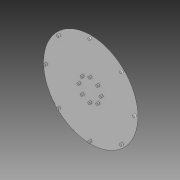
# Autodesk Inventor part: Deskcap
Saved by Autodesk Inventor 2020 (Build 240168000, 168)
## iProperties
Created: 2021-07-12
Part Number: Deskcap
Material: Generic
Document SubType Name: Modeling
Designer: DDeGo
Density: 1 g/cm^3
Appearance: Default
Author: DDeGo
Autodesk Inventor part; units mm, degrees
ref_plane "YZ Plane" through (0, 0, 0) normal (1, 0, 0) x (0, 1, 0)
ref_plane "XZ Plane" through (0, 0, 0) normal (0, 1, 0) x (-1, 0, 0)
ref_plane "XY Plane" through (0, 0, 0) normal (0, 0, 1) x (1, 0, 0)
sketch "Sketch1" plane through (0, 0, 0) normal (0, 0, 1) x (1, 0, 0)
  circle A0 centre (20, 0) radius 2.25
  circle A1 centre (80, 0) radius 2.25
  circle A2 centre (0, 0) radius 85
  line L0 (0, 0) -> (20, 0) construction
  line L1 (20, 0) -> (80, 0) construction
  circle A3 centre (14.1421, 14.1421) radius 2.25
  circle A4 centre (56.5685, 56.5685) radius 2.25
  line L2 (0, 0) -> (14.1421, 14.1421) construction
  line L3 (14.1421, 14.1421) -> (56.5685, 56.5685) construction
  circle A5 centre (0, 20) radius 2.25
  circle A6 centre (0, 80) radius 2.25
  line L4 (0, 0) -> (0, 20) construction
  line L5 (0, 20) -> (0, 80) construction
  circle A7 centre (-14.1421, 14.1421) radius 2.25
  circle A8 centre (-56.5685, 56.5685) radius 2.25
  line L6 (0, 0) -> (-14.1421, 14.1421) construction
  line L7 (-14.1421, 14.1421) -> (-56.5685, 56.5685) construction
  circle A9 centre (-20, 0) radius 2.25
  circle A10 centre (-80, 0) radius 2.25
  line L8 (0, 0) -> (-20, 0) construction
  line L9 (-20, 0) -> (-80, 0) construction
  circle A11 centre (-14.1421, -14.1421) radius 2.25
  circle A12 centre (-56.5685, -56.5685) radius 2.25
  line L10 (0, 0) -> (-14.1421, -14.1421) construction
  line L11 (-14.1421, -14.1421) -> (-56.5685, -56.5685) construction
  circle A13 centre (0, -20) radius 2.25
  circle A14 centre (0, -80) radius 2.25
  line L12 (0, 0) -> (0, -20) construction
  line L13 (0, -20) -> (0, -80) construction
  circle A15 centre (14.1421, -14.1421) radius 2.25
  circle A16 centre (56.5685, -56.5685) radius 2.25
  line L14 (0, 0) -> (14.1421, -14.1421) construction
  line L15 (14.1421, -14.1421) -> (56.5685, -56.5685) construction
  dimension "d0" = 170
  dimension "d1" = 20
  dimension "d2" = 80
  dimension "d3" = 4.5
  dimension "d6" = 360
  constraints: 32 end point, 18 coincident, 17 centre point, 1 collinear, 1 equal radius, 1 horizontal, 71 other
  measures "d0" diameter of A2
  measures "d1" distance of point (0, 0) L0.end
  measures "d2" distance of L1.end point (0, 0)
  measures "d3" diameter of A0
extrude "Extrusion1" add sketch "Sketch1" against normal blind 0.4 contours A0 | A1 | A2 | A3 | A4 | A5 | A6 | A7 | A8 | A9 | A10 | A11 | A12 | A13 | A14 | A15 | A16
extrude "Extrusion2" add sketch "Sketch1" along normal blind 3 contours A0 | A1 | A3 | A4 | A5 | A6 | A7 | A8 | A9 | A10 | A11 | A12 | A13 | A14 | A15 | A16
chamfer "Chamfer1" distance 0.4 angle 45 1 edges at (-85, 0, -0.4)
body "Solid1"
